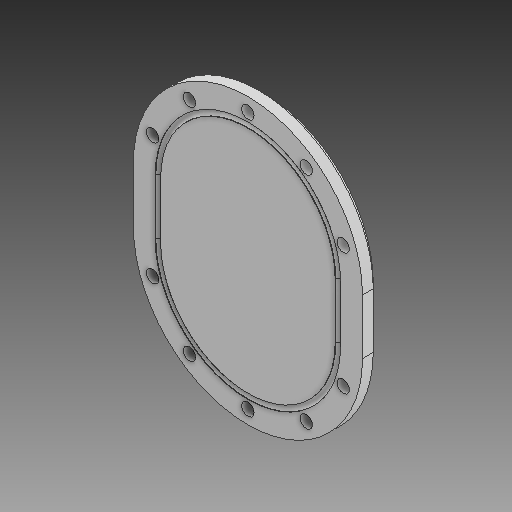
# Autodesk Inventor part: housingPlate
Saved by Autodesk Inventor 2020 (Build 240168000, 168)
## iProperties
Created: 2020-11-25
Part Number: housingPlate
Material: Generic
Document SubType Name: Modeling
Designer: DDeGo
Density: 1 g/cm^3
Appearance: Default
Author: DDeGo
Autodesk Inventor part; units mm, degrees
ref_plane "YZ Plane" through (0, 0, 0) normal (1, 0, 0) x (0, 1, 0)
ref_plane "XZ Plane" through (0, 0, 0) normal (0, 1, 0) x (-1, 0, 0)
ref_plane "XY Plane" through (0, 0, 0) normal (0, 0, 1) x (1, 0, 0)
sketch "Sketch1" plane through (0, 0, 0) normal (0, 0, 1) x (1, 0, 0)
  line L0 (0, 0) -> (0, 5.1) construction
  arc A0 (15.7243, 1.2028) -> (-15.7243, 1.2028) centre (0, 5.1) ccw construction
  line L1 (0, 0) -> (0, -5.1) construction
  arc A1 (-15.7243, -1.2028) -> (15.7243, -1.2028) centre (0, -5.1) ccw construction
  line L2 (0, 5.1) -> (0, -5.1) construction
  line L3 (-21.2, 5.1) -> (-21.2, -5.1)
  line L4 (21.2, -5.1) -> (21.2, 5.1)
  arc A2 (21.2, 5.1) -> (-21.2, 5.1) centre (0, 5.1) ccw
  arc A3 (-21.2, -5.1) -> (21.2, -5.1) centre (0, -5.1) ccw
  arc A4 (-15.7243, -1.2028) -> (-15.7243, 1.2028) centre (-20.5774, 0) ccw construction
  arc A5 (15.7243, 1.2028) -> (15.7243, -1.2028) centre (20.5774, 0) ccw construction
  line L5 (0, 5.1) -> (0, -5.1) construction
  circle A6 centre (0, 0) radius 14.5 construction
  dimension "d0" = 10.2
  dimension "d1" = 16.2
  dimension "d2" = 5
  dimension "d3" = 5
  dimension "d4" = 42.4
  dimension "d8" = 29
  constraints: 16 end point, 12 point on circle, 8 tangent, 7 centre point, 4 coincident, 3 vertical, 2 collinear, 2 equal radius, 2 midpoint, 1 parallel
  measures "d0" distance of L1.end L0.end
  measures "d1" radius of A0
  measures "d2" radial gap between concentric circles of A3 A1
  measures "d3" radius of A4
  measures "d4" distance between parallel lines of L4 L3
  measures "d8" diameter of A6
extrude "Extrusion1" add sketch "Sketch1" along normal blind 3
sketch "Sketch2" plane through (0, 0, 3) normal (0, 0, 1) x (1, 0, 0)
  circle A0 centre (-10.812, -20.3575) radius 1.15 projected
  circle A1 centre (-17.6432, -11.2975) radius 1.15 projected
  circle A2 centre (17.6432, -11.2975) radius 1.15 projected
  circle A3 centre (17.6432, 11.2975) radius 1.15 projected
  circle A4 centre (10.812, -20.3575) radius 1.15 projected
  circle A5 centre (10.812, 20.3575) radius 1.15 projected
  circle A6 centre (-10.812, 20.3575) radius 1.15 projected
  circle A7 centre (0, -23.8) radius 1.15 projected
  circle A8 centre (0, 23.8) radius 1.15 projected
  circle A9 centre (-17.6432, 11.2975) radius 1.15 projected
  circle A10 centre (0, 0) radius 4.075 construction
  arc A11 (-21.1962, -5.5) -> (21.1962, -5.5) centre (0, -5.1) ccw projected
  line L0 (-31.2, -5.5) -> (-21.1962, -5.5) projected
  line L1 (-31.2, 5.5) -> (-31.2, -5.5) projected
  line L2 (-21.1962, 5.5) -> (-31.2, 5.5) projected
  arc A12 (21.1962, 5.5) -> (-21.1962, 5.5) centre (0, 5.1) ccw projected
  line L3 (31.2, 5.5) -> (21.1962, 5.5) projected
  line L4 (31.2, -5.5) -> (31.2, 5.5) projected
  line L5 (21.1962, -5.5) -> (31.2, -5.5) projected
  point P0 (0, 0)
extrude "Extrusion2" cut sketch "Sketch2" against normal through all contours A0 | A1 | A2 | A3 | A4 | A5 | A6 | A7 | A8 | A9
sketch "Sketch5" plane through (0, 0, 3) normal (0, 0, 1) x (1, 0, 0)
  circle A0 centre (10.812, 20.3575) radius 1.15 construction
  circle A1 centre (17.6432, -11.2975) radius 1.15 construction
  circle A2 centre (-10.812, -20.3575) radius 1.15 construction
  circle A3 centre (0, -23.8) radius 1.15 construction
  circle A4 centre (10.812, -20.3575) radius 1.15 construction
  circle A5 centre (17.6432, 11.2975) radius 1.15 construction
  circle A6 centre (-17.6432, -11.2975) radius 1.15 construction
  circle A7 centre (0, 23.8) radius 1.15 construction
  circle A8 centre (-10.812, 20.3575) radius 1.15 construction
  circle A9 centre (-17.6432, 11.2975) radius 1.15 construction
  line L0 (21.2, -5.1) -> (21.2, 5.1) construction
  arc A10 (21.2, 5.1) -> (-21.2, 5.1) centre (0, 5.1) ccw construction
  line L1 (-21.2, 5.1) -> (-21.2, -5.1) construction
  arc A11 (-21.2, -5.1) -> (21.2, -5.1) centre (0, -5.1) ccw construction
  arc A12 (17.15, 5.1) -> (-17.15, 5.1) centre (0, 5.1) ccw
  line L2 (17.15, 5.1) -> (17.15, -5.1)
  arc A13 (-17.15, -5.1) -> (17.15, -5.1) centre (0, -5.1) ccw
  line L3 (-17.15, -5.1) -> (-17.15, 5.1)
  arc A14 (16.15, 5.1) -> (-16.15, 5.1) centre (0, 5.1) ccw
  line L4 (16.15, 5.1) -> (16.15, -5.1)
  arc A15 (-16.15, -5.1) -> (16.15, -5.1) centre (0, -5.1) ccw
  line L5 (-16.15, -5.1) -> (-16.15, 5.1)
  point P0 (0, 0)
  dimension "d20" = 1
  dimension "d21" = 0.4
  constraints: 8 end point, 8 point on circle, 4 centre point, 6 other
  measures "d20" radial gap between concentric circles of A14 A12
extrude "Extrusion5" cut sketch "Sketch5" against normal blind 0.6
fillet "Fillet1" radius 0.5 8 edges at (17.15, 0, 2.4) (0, -22.25, 2.4) (-17.15, 0, 2.4) (0, 22.25, 2.4) (-16.15, 0, 2.4) (0, -21.25, 2.4) (16.15, 0, 2.4) (0, 21.25, 2.4)
chamfer "Chamfer1" distance 1 angle 45 4 edges at (0, -26.3, 0) (21.2, 0, 0) (0, 26.3, 0) (-21.2, 0, 0)
body "Solid1"
